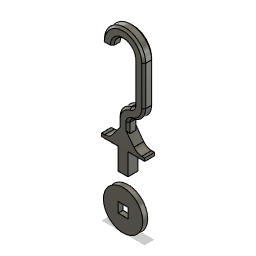
Haken (Autodesk Fusion 360 design; units mm, degrees)
Autodesk Fusion 360 part; units mm, degrees
sketch "Skizze1" plane through (0, 0, 0) normal (0, 1, 0) x (1, 0, 0)
  line L0 (-2.5, 2.5) -> (2.5, 2.5)
  line L1 (2.5, 2.5) -> (2.5, -2.5)
  line L2 (2.5, -2.5) -> (-2.5, -2.5)
  line L3 (-2.5, -2.5) -> (-2.5, 2.5)
  line L4 (-2.5, 2.5) -> (2.5, -2.5) construction
  line L5 (2.5, 2.5) -> (-2.5, -2.5) construction
  dimension "d1" = 5
  constraint horizontal L0
  constraint perpendicular L0 L1
  constraint parallel L0 L2
  constraint parallel L1 L3
  constraint coincident L4 origin
  constraint coincident L5 origin
  constraint equal L0 L1
  measures "d1" distance of L0.start L0.end
extrude "Extrusion1" add sketch "Skizze1" along normal blind 11 makes body 1
sketch "Skizze2" plane through (0, 11, 0) normal (0, 1, 0) x (-1, 0, 0)
  line L0 (2.5, 2.5) -> (-2.5, 2.5)
  line L1 (-2.5, 2.5) -> (-2.5, -2.5)
  line L2 (-2.5, -2.5) -> (2.5, -2.5)
  line L3 (2.5, -2.5) -> (2.5, 2.5)
  line L4 (-11, -2.5) -> (11, -2.5)
  line L5 (11, -2.5) -> (11, 2.5)
  line L6 (11, 2.5) -> (-11, 2.5)
  line L7 (-11, 2.5) -> (-11, -2.5)
  line L8 (-11, -2.5) -> (11, 2.5) construction
  line L9 (11, -2.5) -> (-11, 2.5) construction
  dimension "d4" = 22
  constraint horizontal L4
  constraint perpendicular L4 L5
  constraint parallel L4 L6
  constraint parallel L5 L7
  constraint coincident L8 origin
  constraint coincident L9 origin
  constraint collinear L2 L4
  measures "d4" distance of L4.start L4.end
extrude "Extrusion2" add sketch "Skizze2" along normal blind 1.5 bodies 1
sketch "Skizze3" plane through (0, 0, -2.5) normal (0, 0, -1) x (-1, 0, 0)
  line L0 (-2.5, 0) -> (2.5, 0)
  line L1 (2.5, 0) -> (2.5, 11)
  line L2 (2.5, 11) -> (11, 11)
  line L3 (11, 11) -> (11, 12.5)
  line L4 (11, 12.5) -> (-11, 12.5)
  line L5 (-11, 12.5) -> (-11, 11)
  line L6 (-11, 11) -> (-2.5, 11)
  line L7 (-2.5, 11) -> (-2.5, 0)
  line L8 (-7, 12.5) -> (-2.5, 18.5)
  line L9 (-2.5, 18.5) -> (2.5, 18.5)
  line L10 (2.5, 18.5) -> (7, 12.5)
  line L11 (0, 18.5) -> (0, 12.5) construction
  dimension "d7" = 6
  dimension "d8" = 14
  constraint coincident L4 L8.start
  constraint parallel L4 L9
  constraint coincident L4 L10.end
  constraint midpoint L9 L11.start
  constraint midpoint L4 L11.end
  constraint vertical L11
  constraint symmetric L8 L10 L11
  constraint coincident L1 L9.end
  measures "d7" distance of L4 L9
  measures "d8" distance of L8.start L10.end
extrude "Extrusion3" add sketch "Skizze3" against normal blind 5 contours L4 L8 L9 L10 bodies 1
sketch "Skizze4" plane through (0, 0, 0) normal (0, 0, 1) x (1, 0, 0)
  line L0 (0, 18.5) -> (0, 23.5)
  arc A0 (3.9024, 28.378) -> (0, 23.5) centre (5, 23.5) ccw
  arc A1 (3.9024, 28.378) -> (8, 33.5) centre (2.75, 33.5) ccw
  line L1 (8, 33.5) -> (8, 53.5)
  arc A2 (8, 53.5) -> (-8, 53.5) centre (0, 53.5) ccw
  line L2 (2.5, 18.5) -> (-2.5, 18.5)
  dimension "d11" = 2.5
  dimension "d12" = 5
  dimension "d13" = 20
  dimension "d14" = 8
  dimension "d15" = 5
  dimension "d16" = 15
  constraint vertical L0
  constraint tangent L0 A0
  constraint tangent A0 A1
  constraint parallel L0 L1
  constraint tangent L1 A2
  constraint horizontal L1.end A2.end
  constraint coincident L0 A2.centre
  constraint tangent A1 L1
  constraint coincident L0.start L2
  measures "d11" distance of L0.start L2.end
  measures "d12" distance of L0.start L0.end
  measures "d13" distance of A1.end L1.end
  measures "d14" radius of A2
  measures "d15" radius of A0
  measures "d16" distance of A1.centre L2
sweep "Sweeping1" add 1 faces at (0.8333, 18.5, -0.8333) path "Skizze4" along L0 A0 A1 L1 A2 on bodies 1 bodies 1
chamfer "Fase1" distance 1 angle 45 20 edges at (-0.8565, 28.1852, 2.5) (4.8974, 31.7821, 2.5) (5.5, 43.5, 2.5) (0, 59, 2.5) (-2.5, 21, 2.5) (8.8017, 28.6586, 2.5) (10.5, 43.5, 2.5) (0, 64, 2.5) (2.5, 21, 2.5) (3.0478, 25.0617, 2.5) (-0.8565, 28.1852, -2.5) (4.8974, 31.7821, -2.5) (5.5, 43.5, -2.5) (0, 59, -2.5) (-2.5, 21, -2.5) (3.0478, 25.0617, -2.5) (8.8017, 28.6586, -2.5) (10.5, 43.5, -2.5) (0, 64, -2.5) (2.5, 21, -2.5) on bodies 1
sketch "Skizze5" plane through (0, 0, 0) normal (0, 0, 1) x (1, 0, 0)
  circle A0 centre (0, -16) radius 10
  line L0 (-2.55, -13.45) -> (2.55, -13.45)
  line L1 (2.55, -13.45) -> (2.55, -18.55)
  line L2 (2.55, -18.55) -> (-2.55, -18.55)
  line L3 (-2.55, -18.55) -> (-2.55, -13.45)
  line L4 (-2.55, -13.45) -> (2.55, -18.55) construction
  line L5 (2.55, -13.45) -> (-2.55, -18.55) construction
  point P0 (0, -16)
  dimension "d24" = 20
  dimension "d25" = 5.1
  dimension "d26" = 16
  constraint horizontal L0
  constraint perpendicular L0 L1
  constraint parallel L0 L2
  constraint parallel L1 L3
  constraint coincident L4 P0
  constraint coincident L5 P0
  constraint coincident P0 A0.centre
  constraint equal L0 L3
  constraint vertical origin A0.centre
  measures "d24" diameter of A0
  measures "d25" distance of L0.start L0.end
  measures "d26" distance of origin A0.centre
extrude "Extrusion4" add sketch "Skizze5" along normal up to surface (2.5 mm away) separate body makes body 2
fillet "Abrundung1" radius 5 2 edges at (-7, 12.5, 0) (7, 12.5, 0) on bodies 1
